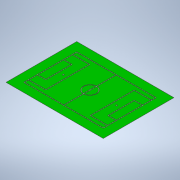
# Autodesk Inventor part: SoccerField_KidSize
Saved by Autodesk Inventor 2022 (Build 260153000, 153)
## iProperties
Created: 2022-10-30
Part Number: SoccerField_KidSize
Material: 一般
Document SubType Name: Modeling
Designer: Masato Kubotera
Density: 1 g/cm^3
Appearance: 既定
Author: Masato Kubotera
Autodesk Inventor part; units mm, degrees
ref_plane "YZ Plane" through (0, 0, 0) normal (1, 0, 0) x (0, 1, 0)
ref_plane "XZ Plane" through (0, 0, 0) normal (0, 1, 0) x (-1, 0, 0)
ref_plane "XY Plane" through (0, 0, 0) normal (0, 0, 1) x (1, 0, 0)
sketch "スケッチ1" plane through (0, 0, 0) normal (0, 0, 1) x (1, 0, 0)
  line L0 (-5500, -4000) -> (5500, -4000)
  line L1 (5500, -4000) -> (5500, 4000)
  line L2 (5500, 4000) -> (-5500, 4000)
  line L3 (-5500, 4000) -> (-5500, -4000)
  line L4 (-5500, -4000) -> (5500, 4000) construction
  line L5 (5500, -4000) -> (-5500, 4000) construction
  line L6 (5500, 0) -> (-5500, 0) construction
  line L7 (0, 4000) -> (0, -4000)
  line L8 (-4450, -2950) -> (4450, -2950)
  line L9 (4450, -2950) -> (4450, -2500)
  line L10 (4450, 2950) -> (-4450, 2950)
  line L11 (-4450, 2950) -> (-4450, -2950)
  line L12 (-4450, -2950) -> (4450, 2950) construction
  line L13 (4450, -2950) -> (-4450, 2950) construction
  line L14 (-4500, -3000) -> (4500, -3000)
  line L15 (4500, -3000) -> (4500, 1400)
  line L16 (4500, 3000) -> (-4500, 3000)
  line L17 (-4500, 3000) -> (-4500, -3000)
  line L18 (-4500, -3000) -> (4500, 3000) construction
  line L19 (4500, -3000) -> (-4500, 3000) construction
  line L20 (-4475, -2975) -> (4475, -2975) construction
  line L21 (4475, -2975) -> (4475, 2975) construction
  line L22 (4475, 2975) -> (-4475, 2975) construction
  line L23 (-4475, 2975) -> (-4475, -2975) construction
  line L24 (-4475, -2975) -> (4475, 2975) construction
  line L25 (4475, -2975) -> (-4475, 2975) construction
  line L26 (4475, 1350) -> (5100, 1350) construction
  line L27 (5100, 1350) -> (5100, -1350) construction
  line L28 (4500, 1300) -> (5050, 1300)
  line L29 (5050, 1300) -> (5050, -1300)
  line L30 (4500, 1400) -> (5050, 1400)
  line L31 (5150, 1400) -> (5150, -1400)
  line L32 (4475, -1350) -> (5100, -1350) construction
  line L33 (4500, -1300) -> (5050, -1300)
  line L34 (4500, -1400) -> (5150, -1400)
  line L35 (4475, 1475) -> (3525, 1475) construction
  line L36 (3525, 1475) -> (3525, -1475) construction
  line L37 (3525, -1475) -> (4475, -1475) construction
  line L38 (4450, 1500) -> (3500, 1500)
  line L39 (3500, 1500) -> (3500, -1500)
  line L40 (3500, -1500) -> (4450, -1500)
  line L41 (4450, -1450) -> (3550, -1450)
  line L42 (3550, -1450) -> (3550, 1450)
  line L43 (3550, 1450) -> (4450, 1450)
  line L44 (4475, 2475) -> (2525, 2475) construction
  line L45 (2525, 2475) -> (2525, -2475) construction
  line L46 (4450, 2500) -> (2500, 2500)
  line L47 (2500, 2500) -> (2500, -2500)
  line L48 (4450, 2450) -> (2550, 2450)
  line L49 (2550, 2450) -> (2550, -2450)
  line L50 (4450, -2500) -> (2500, -2500)
  line L51 (4450, -2450) -> (2550, -2450)
  line L52 (4475, -2475) -> (2525, -2475) construction
  arc A0 (25, 699.5534) -> (-25, 699.5534) centre (0, 0) ccw construction
  arc A1 (25, 749.5832) -> (-25, 749.5832) centre (0, 0) ccw construction
  line L53 (25, 2950) -> (25, 749.5832)
  line L54 (-25, 2950) -> (-25, 749.5832)
  line L55 (-75, 25) -> (-25, 25)
  line L56 (75, 25) -> (75, -25)
  line L57 (75, -25) -> (25, -25)
  line L58 (-75, -25) -> (-75, 25)
  line L59 (-75, 25) -> (75, -25) construction
  line L60 (75, 25) -> (-75, -25) construction
  line L61 (2925, 25) -> (2975, 25)
  line L62 (3075, 25) -> (3075, -25)
  line L63 (3075, -25) -> (3025, -25)
  line L64 (2925, -25) -> (2925, 25)
  line L65 (2925, 25) -> (3075, -25) construction
  line L66 (3075, 25) -> (2925, -25) construction
  line L67 (2975, 75) -> (3025, 75)
  line L68 (3025, 75) -> (3025, 25)
  line L69 (3025, -75) -> (2975, -75)
  line L70 (2975, -75) -> (2975, -25)
  line L71 (2975, 75) -> (3025, -75) construction
  line L72 (3025, 75) -> (2975, -75) construction
  line L73 (4450, 2450) -> (4450, 2500) construction
  line L74 (4450, 2500) -> (4450, 2950)
  line L75 (4450, 1450) -> (4450, 1500) construction
  line L76 (4450, 1500) -> (4450, 2450)
  line L77 (5050, 1400) -> (5150, 1400)
  line L78 (4500, 1400) -> (4500, 3000)
  line L79 (4450, -1500) -> (4450, -1450) construction
  line L80 (4450, -1450) -> (4450, 1450)
  line L81 (4450, -2500) -> (4450, -2450) construction
  line L82 (4450, -2450) -> (4450, -1500)
  line L83 (2975, -25) -> (2975, 25) construction
  line L84 (2975, 25) -> (3025, 25) construction
  line L85 (3025, 25) -> (3025, -25) construction
  line L86 (3025, -25) -> (3025, -75)
  line L87 (3025, 25) -> (3075, 25)
  line L88 (2975, -25) -> (2925, -25)
  line L89 (2975, 25) -> (2975, 75)
  line L90 (3025, -25) -> (2975, -25) construction
  arc A2 (566.1153, 411.7202) -> (25, 699.5534) centre (0, 0) ccw
  arc A3 (25, -749.5832) -> (25, 749.5832) centre (0, 0) ccw
  line L91 (25, 699.5534) -> (25, 25)
  line L92 (25, 749.5832) -> (25, 699.5534) construction
  line L93 (-25, 699.5534) -> (-25, 25)
  arc A4 (-25, 749.5832) -> (-25, -749.5832) centre (0, 0) ccw
  line L94 (-25, 749.5832) -> (-25, 699.5534) construction
  line L95 (-25, 25) -> (-25, -25) construction
  arc A5 (-25, 699.5534) -> (-25, -699.5534) centre (0, 0) ccw
  line L96 (25, -699.5534) -> (25, -749.5832) construction
  arc A6 (-25, -699.5534) -> (25, -699.5534) centre (0, 0) ccw construction
  arc A7 (-25, -749.5832) -> (25, -749.5832) centre (0, 0) ccw construction
  line L97 (25, -749.5832) -> (25, -2950)
  line L98 (-25, -749.5832) -> (-25, -2950)
  line L99 (-25, -699.5534) -> (-25, -749.5832) construction
  arc A8 (25, -699.5534) -> (566.1153, 411.7202) centre (0, 0) ccw
  line L100 (-25, 25) -> (0, 25) construction
  line L101 (0, 25) -> (25, 25) construction
  line L102 (25, 25) -> (25, -25) construction
  line L103 (25, 25) -> (75, 25)
  line L104 (25, -25) -> (-25, -25) construction
  line L105 (25, -25) -> (25, -699.5534)
  line L106 (-25, -25) -> (-25, -699.5534)
  line L107 (-25, -25) -> (-75, -25)
  point P0 (3000, 0)
  point P1 (452.5, -127.5)
  point P2 (447.5, -247.5)
  point P3 (302.5, -2.5)
  point P4 (297.5, -2.5)
  point P5 (297.5, 2.5)
  point P6 (302.5, 2.5)
  point P7 (2.5, 77.4597)
  point P8 (2.5, -77.4597)
  point P9 (447.5, -252.5)
  point P10 (2.5, -2.5)
  point P11 (25, 724.5688)
  point P12 (2.5, 72.4569)
  point P13 (2.5, 2.5)
  point P14 (-2.5, 2.5)
  point P15 (-2.5, 72.4569)
  point P16 (-25, 724.5688)
  point P17 (-2.5, -2.5)
  point P18 (-2.5, 77.4597)
  point P19 (-2.5, 77.4597)
  point P20 (452.5, -132.5)
  point P21 (606.5521, 441.1288)
  point P22 (0, 3000)
  point P23 (0, -3000)
  point P24 (0, -2950)
  point P25 (0, 2950)
  dimension "d2" = 50
  dimension "d3" = 50
  dimension "d8" = 100
  dimension "d9" = 100
  dimension "d11" = 50
  dimension "d12" = 50
  dimension "d15" = 50
  dimension "d16" = 50
  dimension "d20" = 50
  dimension "d22" = 50
  dimension "d23" = 50
  dimension "d24" = 150
  dimension "d25" = 50
  dimension "d26" = 50
  dimension "d27" = 150
  dimension "d28" = 150
  dimension "d34" = 2600
  dimension "d35" = 1000
  dimension "d36" = 1000
  dimension "d37" = 2000
  dimension "d38" = 5000
  dimension "d39" = 1500
  dimension "d40" = 1000
  dimension "d41" = 6000
  dimension "d42" = 9000
  dimension "d43" = 3000
  dimension "d45" = 600
  dimension "d46" = 1500
  constraints: 216 end point, 78 perpendicular, 53 parallel, 20 point on circle, 19 point on line, 18 midpoint, 16 horizontal, 12 symmetric about line, 9 centre point, 2 coincident, 12 other
  measures "d2" distance between parallel lines of L9 L15
  measures "d3" distance between parallel lines of L16 L10
  measures "d8" distance between parallel lines of L29 L31
  measures "d9" distance between parallel lines of L30 L28
  measures "d11" distance between parallel lines of L38 L43
  measures "d12" distance between parallel lines of L39 L42
  measures "d15" distance between parallel lines of L48 L46
  measures "d16" distance between parallel lines of L47 L49
  measures "d20" radial gap between concentric circles of A1 A0
  measures "d22" distance between parallel lines of L54 L53
  measures "d23" distance of L56.start L56.end
  measures "d24" distance of L56.end L58.start
  measures "d25" distance of L62.start L62.end
  measures "d26" distance of L69.start L69.end
  measures "d27" distance of L62.end L64.start
  measures "d28" distance of L69.end L67.start
  measures "d34" distance between parallel lines of L28 L33
  measures "d35" distance between parallel lines of L2 L16
  measures "d36" distance between parallel lines of L1 L78
  measures "d37" distance between parallel lines of L78 L47
  measures "d38" distance between parallel lines of L50 L46
  measures "d39" distance from line of L15 point (3000, 0)
  measures "d40" distance between parallel lines of L78 L39
  measures "d41" distance between parallel lines of L16 L14
  measures "d42" distance between parallel lines of L78 L17
  measures "d43" distance between parallel lines of L40 L38
  measures "d45" distance between parallel lines of L29 L76
  measures "d46" diameter of A3
extrude "押し出し1" add sketch "スケッチ1" along normal blind 3 contours L7 L14 L15 L34 L31 L77 L30 L78 L16 L2 L1 L0 | L97 A3 L53 L10 L74 L46 L47 L50 L9 L8 | L15 L33 L29 L28 L30 L77 L31 L34 | L15 L28 L29 L33 | L38 L39 L40 L82 L51 L49 L48 L76 | L41 L42 L43 L80 | L103 L91 A2 A8 L105 L57 L56
extrude "押し出し2" add sketch "スケッチ1" along normal blind 3 separate body contours L7 L8 L9 L50 L47 L46 L74 L10 L16 L78 L15 L14 | L8 L98 A4 L54 L10 L7 | L7 L10 L53 A3 L97 L8 | L61 L89 L67 L68 L87 L62 L63 L86 L69 L70 L88 L64
mirror "ミラー1" about plane through (0, 0, 0) normal (1, 0, 0) bodies 2 1
equation "\"d3\" = d2"
equation "\"d11\" = d2"
equation "\"d12\" = d2"
equation "\"d15\" = d2"
equation "\"d16\" = d2"
equation "\"d20\" = d2"
equation "\"d22\" = d2"
equation "\"d23\" = d2"
equation "\"d24\" = 3 * d23"
equation "\"d25\" = d2"
equation "\"d26\" = d2"
equation "\"d27\" = d24"
equation "\"d28\" = d24"
